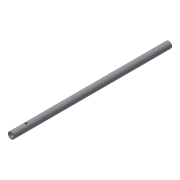
# Autodesk Inventor part: transmission tube v1
Saved by Autodesk Inventor 2014 (Build 180170000, 170)
## iProperties
Created: 2014-02-22
Part Number: transmission tube v1
Material: Generic
Document SubType Name: Modeling
Designer: Owner
Density: 1 g/cm^3
Appearance: Default
Author: Owner
Autodesk Inventor part; units mm, degrees
sketch "Sketch1" plane through (0, 0, 0) normal (0, 0, 1) x (1, 0, 0)
  circle A0 centre (0, 0) radius 6.35
  circle A1 centre (0, 0) radius 3.937
  dimension "d0" = 12.7
  dimension "d1" = 2.413
  constraints: 2 centre point, 2 coincident
  measures "d0" diameter of A0
  measures "d1" radial gap between concentric circles of A0 A1
extrude "Extrusion1" add sketch "Sketch1" against normal blind 304.8
ref_plane "Work Plane1" through (0, 0, -28.575) normal (0, 0, 1) x (1, 0, 0)
sketch "Sketch2" plane through (0, 0, -28.575) normal (0, 0, 1) x (1, 0, 0)
  circle A0 centre (0, 0) radius 6.35 projected
  line L0 (0, 0) -> (5.4993, -3.175) construction
  line L1 (0, 0) -> (0, 6.35) construction
  line L2 (0, 0) -> (-5.4993, -3.175) construction
  dimension "d6" = 120
  dimension "d7" = 120
  constraints: 6 end point, 3 point on circle, 1 vertical
  measures "d6" angle of L0 L1
  measures "d7" angle of L2 L0
ref_plane "Work Plane2" through (0, 6.35, -28.575) normal (0, 1, 0) x (-1, 0, 0)
sketch "Sketch3" plane through (0, 6.35, -28.575) normal (0, 1, 0) x (-1, 0, 0)
  circle A0 centre (0, 0) radius 2.3813
  dimension "d8" = 4.7625
  constraints: 1 centre point
  measures "d8" diameter of A0
extrude "Extrusion2" cut sketch "Sketch3" against normal up to next
ref_plane "Work Plane3" through (5.4993, -3.175, -28.575) normal (0.866, -0.5, 0) x (0.5, 0.866, 0)
sketch "Sketch4" plane through (5.4993, -3.175, -28.575) normal (0.866, -0.5, 0) x (0.5, 0.866, 0)
  circle A0 centre (0, 0) radius 2.3813
  dimension "d11" = 4.7625
  constraints: 1 centre point, 1 coincident
  measures "d11" diameter of A0
extrude "Extrusion3" cut sketch "Sketch4" against normal up to next
ref_plane "Work Plane4" through (-5.4993, -3.175, -28.575) normal (-0.866, -0.5, 0) x (0.5, -0.866, 0)
sketch "Sketch5" plane through (-5.4993, -3.175, -28.575) normal (-0.866, -0.5, 0) x (0.5, -0.866, 0)
  circle A0 centre (0, 0) radius 2.3812
  dimension "d14" = 4.7625
  constraints: 1 centre point, 1 coincident
  measures "d14" diameter of A0
extrude "Extrusion4" cut sketch "Sketch5" against normal up to next
body "Solid1"
